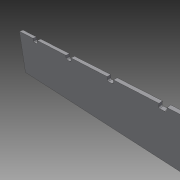
# Autodesk Inventor part: front_panel_bottom
Saved by Autodesk Inventor 2014 (Build 180170000, 170)
## iProperties
Created: 2014-03-23
Part Number: front_panel_bottom
Material: Generic
Document SubType Name: Modeling
Designer: buben
Density: 1 g/cm^3
Appearance: Default
Author: buben
Autodesk Inventor part; units mm, degrees
ref_plane "YZ Plane" through (0, 0, 0) normal (1, 0, 0) x (0, 1, 0)
ref_plane "XZ Plane" through (0, 0, 0) normal (0, 1, 0) x (-1, 0, 0)
ref_plane "XY Plane" through (0, 0, 0) normal (0, 0, 1) x (1, 0, 0)
sketch "Sketch1" plane through (0, 0, 0) normal (0, 1, 0) x (-1, 0, 0)
  line L0 (0, 0) -> (-300, 0)
  line L1 (-300, 0) -> (-300, -74.151)
  line L2 (-300, -74.151) -> (0, -74.151)
  line L3 (0, -74.151) -> (0, 0)
  dimension "d0" = 300
  dimension "d1" = 74.151
  constraints: 8 end point, 2 parallel, 1 horizontal, 1 perpendicular
  measures "d0" distance of L0.start L0.end
  measures "d1" distance of L2.end L0.start
extrude "Extrusion1" add sketch "Sketch1" along normal blind 6.5
sketch "Sketch2" plane through (0, 6.5, 0) normal (0, 1, 0) x (1, 0, 0)
  line L0 (0, 0) -> (300, 0) projected
  line L1 (300, 74.151) -> (0, 74.151) projected
  line L2 (150, 74.151) -> (150, 0) construction
  line L3 (34.711, 0) -> (44.711, 0)
  line L4 (44.711, 0) -> (44.711, 4)
  line L5 (42.711, 6) -> (36.711, 6)
  line L6 (34.711, 4) -> (34.711, 0)
  line L7 (107.911, 0) -> (117.911, 0)
  line L8 (117.911, 0) -> (117.911, 4)
  line L9 (115.911, 6) -> (109.911, 6)
  line L10 (107.911, 4) -> (107.911, 0)
  arc A0 (36.711, 6) -> (34.711, 4) centre (36.711, 4) ccw
  arc A1 (44.711, 4) -> (42.711, 6) centre (42.711, 4) ccw
  arc A2 (109.911, 6) -> (107.911, 4) centre (109.911, 4) ccw
  arc A3 (117.911, 4) -> (115.911, 6) centre (115.911, 4) ccw
  line L11 (265.289, 0) -> (255.289, 0)
  line L12 (255.289, 0) -> (255.289, 4)
  line L13 (257.289, 6) -> (263.289, 6)
  line L14 (265.289, 4) -> (265.289, 0)
  line L15 (192.089, 0) -> (182.089, 0)
  line L16 (182.089, 0) -> (182.089, 4)
  line L17 (184.089, 6) -> (190.089, 6)
  line L18 (192.089, 4) -> (192.089, 0)
  arc A4 (265.289, 4) -> (263.289, 6) centre (263.289, 4) ccw
  arc A5 (257.289, 6) -> (255.289, 4) centre (257.289, 4) ccw
  arc A6 (192.089, 4) -> (190.089, 6) centre (190.089, 4) ccw
  arc A7 (184.089, 6) -> (182.089, 4) centre (184.089, 4) ccw
  point P0 (39.711, 6)
  point P1 (112.911, 6)
  point P2 (260.289, 6)
  point P3 (187.089, 6)
  dimension "d10" = 2
  dimension "d11" = 73.2
  dimension "d12" = 37.089
  dimension "d13" = 10
  dimension "d14" = 10
  dimension "d15" = 6
  constraints: 34 end point, 18 symmetric about line, 16 point on circle, 8 centre point, 8 tangent, 4 midpoint, 4 parallel, 3 equal radius, 2 horizontal, 2 perpendicular, 2 point on line, 1 collinear, 4 other
  measures "d10" radius of A0
  measures "d11" distance of point (112.911, 6) point (39.711, 6)
  measures "d12" distance from line of L2 point (112.911, 6)
  measures "d13" distance between parallel lines of L6 L4
  measures "d14" distance between parallel lines of L8 L10
  measures "d15" distance between parallel lines of L0 L5
extrude "Extrusion2" cut sketch "Sketch2" against normal through all
equation "\"d13\" = d14"
body "Solid1"
